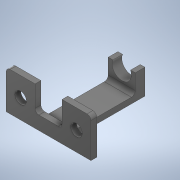
# Autodesk Inventor part: TempSensorHolder
Saved by Autodesk Inventor 2020 (Build 240168000, 168)
## iProperties
Created: 2020-05-16
Part Number: TempSensorHolder
Material: Типовые
Document SubType Name: Modeling
Designer: Михаил
Density: 1 g/cm^3
Appearance: По умолчанию
Author: Михаил
Autodesk Inventor part; units mm, degrees
ref_plane "YZ Plane" through (0, 0, 0) normal (1, 0, 0) x (0, 1, 0)
ref_plane "XZ Plane" through (0, 0, 0) normal (0, 1, 0) x (-1, 0, 0)
ref_plane "XY Plane" through (0, 0, 0) normal (0, 0, 1) x (1, 0, 0)
sketch "Эскиз1" plane through (0, 0, 0) normal (0, 1, 0) x (-1, 0, 0)
  line L0 (0, 0) -> (14, 0)
  line L1 (14, 0) -> (14, -43)
  line L2 (14, -43) -> (0, -43)
  line L3 (0, -43) -> (0, 0)
  dimension "d1" = 43
  dimension "d2" = 14
  constraints: 8 end point, 2 parallel, 1 horizontal, 1 perpendicular
  measures "d1" distance of L0.end L1.end
  measures "d2" distance of L1.end L2.end
extrude "Выдавливание1" add sketch "Эскиз1" along normal blind 3
sketch "Эскиз2" plane through (-14, 0, 0) normal (0, 0, 1) x (1, 0, 0)
  line L0 (0, 0) -> (0, 3) projected
  line L1 (0, 0) -> (-15, 0)
  line L2 (-15, 0) -> (-15, 20)
  line L3 (-15, 20) -> (0, 20)
  line L4 (0, 20) -> (0, 0)
  line L5 (14, 0) -> (0, 0) projected
  line L6 (14, 0) -> (29, 0)
  line L7 (29, 0) -> (29, 20)
  line L8 (29, 20) -> (14, 20)
  line L9 (14, 20) -> (14, 0)
  dimension "d5" = 15
  dimension "d6" = 20
  dimension "d7" = 15
  dimension "d8" = 20
  constraints: 16 end point, 4 parallel, 2 horizontal, 2 perpendicular
  measures "d5" distance of L2.end L3.end
  measures "d6" distance of L1.end L2.end
  measures "d7" distance of L8.end L7.end
  measures "d8" distance of L7.end L6.end
extrude "Выдавливание2" add sketch "Эскиз2" against normal blind 3
sketch "Эскиз3" plane through (0, 3, 0) normal (0, 1, 0) x (1, 0, 0)
  line L0 (-14, 43) -> (-14, 3) projected
  line L1 (0, 0) -> (-14, 0)
  line L2 (-14, 0) -> (-14, 3)
  line L3 (-14, 3) -> (0, 3)
  line L4 (0, 3) -> (0, 0)
  constraints: 8 end point, 2 parallel, 1 horizontal, 1 perpendicular
extrude "Выдавливание3" add sketch "Эскиз3" along normal blind 4
fillet "Сопряжение1" radius 2 4 edges at (-14, 7, -1.5) (0, 7, -1.5) (15, 20, -1.5) (-29, 20, -1.5)
fillet "Сопряжение2" radius 2 1 edges at (-7, 3, -3)
sketch "Эскиз5" plane through (0, 3, 0) normal (0, 1, 0) x (1, 0, 0)
  line L0 (0, 5) -> (0, 43) projected
  line L1 (0, 43) -> (-14, 43)
  line L2 (-14, 43) -> (-14, 38)
  line L3 (-14, 38) -> (0, 38)
  line L4 (0, 38) -> (0, 43)
  point P0 (0, 0)
  point P1 (0, 38)
  dimension "d21" = 14
  dimension "d22" = 5
  constraints: 8 end point, 2 parallel, 1 horizontal, 1 perpendicular
  measures "d21" distance of L3.end L2.end
  measures "d22" distance of L2.end L1.end
extrude "Выдавливание5" add sketch "Эскиз5" along normal blind 10
sketch "Эскиз6" plane through (0, 0, -43) normal (0, 0, -1) x (-1, 0, 0)
  circle A0 centre (7, 11) radius 5
  line L0 (0, 0) -> (14, 0) projected
  line L1 (0, 13) -> (14, 13) projected
  line L2 (0, 0) -> (0, 13) projected
  point P0 (11.5826, 13)
  point P1 (2.4174, 13)
  dimension "d25" = 10
  dimension "d27" = 2
  dimension "d28" = 7
  constraints: 1 centre point
  measures "d25" diameter of A0
  measures "d27" distance from line of L1 A0.centre
  measures "d28" distance from line of L2 A0.centre
extrude "Выдавливание6" cut sketch "Эскиз6" against normal blind 7 contours A0 L1 picked at (7.9729, 10.9801)
fillet "Сопряжение3" radius 2 1 edges at (-7, 3, -38)
fillet "Сопряжение4" radius 2 2 edges at (0, 2.5, -3) (-14, 2.5, -3)
sketch "Эскиз7" plane through (-14, 0, -3) normal (0, 0, -1) x (-1, 0, 0)
  circle A0 centre (-21.5, 10) radius 3
  line L0 (-14, 9) -> (-14, 20) projected
  line L1 (-29, 0) -> (-16, 0) projected
  circle A1 centre (7.5, 10) radius 3
  line L2 (0, 20) -> (0, 9) projected
  line L3 (2, 0) -> (15, 0) projected
  point P0 (-14, 0)
  dimension "d33" = 6
  dimension "d34" = 7.5
  dimension "d35" = 10
  dimension "d36" = 6
  dimension "d37" = 7.5
  dimension "d38" = 10
  constraints: 2 centre point
  measures "d33" diameter of A0
  measures "d34" distance from line of L0 A0.centre
  measures "d35" distance from line of L1 A0.centre
  measures "d36" diameter of A1
  measures "d37" distance from line of L2 A1.centre
  measures "d38" distance from line of L3 A1.centre
extrude "Выдавливание7" cut sketch "Эскиз7" against normal blind 10
